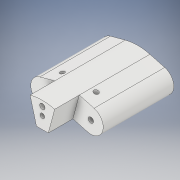
# Autodesk Inventor part: Body
Saved by Autodesk Inventor 2017 SP1 (Build 210196100, 196)
## iProperties
Created: 2018-02-11
Part Number: Body
Material: ABS Plastic
Document SubType Name: Modeling
Designer: Zach
Density: 1.06 g/cm^3
Appearance: CR White
Author: Zach
Autodesk Inventor part; units mm, degrees
ref_plane "YZ Plane" through (0, 0, 0) normal (1, 0, 0) x (0, 1, 0)
ref_plane "XZ Plane" through (0, 0, 0) normal (0, 1, 0) x (-1, 0, 0)
ref_plane "XY Plane" through (0, 0, 0) normal (0, 0, 1) x (1, 0, 0)
sketch "Sketch1" plane through (0, 0, 0) normal (0, 0, 1) x (1, 0, 0)
  circle A0 centre (31.1774, 0) radius 8 construction
  circle A1 centre (0, 0) radius 8 construction
  line L0 (7.5887, 10.3156) -> (11.7298, -5.1392) construction
  line L1 (11.7298, -5.1392) -> (2.0706, -7.7274)
  line L2 (-2.0706, 7.7274) -> (7.5887, 10.3156)
  line L3 (19.4476, -5.1392) -> (23.5887, 10.3156) construction
  line L4 (23.5887, 10.3156) -> (33.248, 7.7274)
  line L5 (19.4476, -5.1392) -> (29.1069, -7.7274)
  line L6 (7.5887, 10.3156) -> (23.5887, 10.3156) construction
  line L7 (11.7298, -5.1392) -> (19.4476, -5.1392)
  arc A2 (-2.0706, 7.7274) -> (2.0706, -7.7274) centre (0, 0) ccw
  arc A3 (29.1069, -7.7274) -> (33.248, 7.7274) centre (31.1774, 0) ccw
  arc A4 (23.5887, 10.3156) -> (7.5887, 10.3156) centre (15.5887, -19.5408) ccw
  point P0 (15.5887, 10.3156)
  dimension "d0" = 16
  dimension "d1" = 16
  dimension "d2" = 16
  dimension "d3" = 10
  dimension "d4" = 10
  dimension "d5" = 16
  dimension "d6" = 16
  dimension "d7" = 75
  constraints: 16 end point, 10 point on circle, 10 tangent, 5 centre point, 2 horizontal alignment, 2 perpendicular, 1 coincident, 1 horizontal, 1 midpoint, 1 point on line
  measures "d0" diameter of A0
  measures "d1" diameter of A1
  measures "d2" distance of L0.start L7.start
  measures "d3" distance from line of A1.centre L0
  measures "d4" distance from line of L3 A0.centre
  measures "d5" distance of L5.start L3.end
  measures "d6" distance of L0.start L3.end
  measures "d7" angle of L6 L0
extrude "Extrusion1" add sketch "Sketch1" along normal blind 46
sketch "Sketch2" plane through (0, 0, 46) normal (0, 0, 1) x (1, 0, 0)
  arc A0 (-2.0706, 7.7274) -> (2.0706, -7.7274) centre (0, 0) ccw projected
  arc A1 (29.1069, -7.7274) -> (33.248, 7.7274) centre (31.1774, 0) ccw projected
  line L0 (11.7298, -5.1392) -> (19.4476, -5.1392) projected
  circle A2 centre (0, 0) radius 1.75
  circle A3 centre (31.1774, 0) radius 1.75
  circle A4 centre (15.5887, 7.8608) radius 1.75
  point P0 (0, 0)
  point P1 (15.5887, -5.1392)
  dimension "d11" = 3.5
  dimension "d12" = 3.5
  dimension "d13" = 3.5
  dimension "d14" = 13
  constraints: 3 centre point, 2 coincident, 1 midpoint, 1 vertical alignment
  measures "d11" diameter of A2
  measures "d12" diameter of A3
  measures "d13" diameter of A4
  measures "d14" distance from line of L0 A4.centre
extrude "Extrusion2" cut sketch "Sketch2" against normal through all
sketch "Sketch3" plane through (0, 0, 46) normal (0, 0, 1) x (1, 0, 0)
  arc A0 (23.5887, 10.3156) -> (7.5887, 10.3156) centre (15.5887, -19.5408) ccw projected
  line L0 (7.5887, 10.3156) -> (23.5887, 10.3156)
  line L1 (19.4476, -5.1392) -> (29.1069, -7.7274) projected
  line L2 (23.5887, 10.3156) -> (19.4476, -5.1392)
  line L3 (11.7298, -5.1392) -> (19.4476, -5.1392) projected
  line L4 (19.4476, -5.1392) -> (11.7298, -5.1392)
  line L5 (11.7298, -5.1392) -> (7.5887, 10.3156)
  circle A1 centre (15.5887, 7.8608) radius 1.75 projected
  point P0 (0, 0)
  constraints: 8 end point, 1 collinear, 1 horizontal, 1 perpendicular
extrude "Extrusion3" add sketch "Sketch3" along normal blind 16
sketch "Sketch4" plane through (0, 0, 62) normal (0, 0, 1) x (1, 0, 0)
  arc A0 (23.5887, 10.3156) -> (7.5887, 10.3156) centre (15.5887, -19.5408) ccw construction
  line L0 (7.5887, 10.3156) -> (23.5887, 10.3156) construction
  line L1 (23.5887, 10.3156) -> (15.5887, 10.3156) construction
  line L2 (11.7298, -5.1392) -> (19.4476, -5.1392) construction
  line L3 (15.5887, -5.1392) -> (15.5887, 10.3156) construction
  circle A1 centre (15.5887, 2.5882) radius 1.5
  point P0 (0, 0)
  dimension "d19" = 3
  constraints: 6 end point, 3 midpoint, 1 centre point, 1 horizontal, 1 perpendicular
  measures "d19" diameter of A1
extrude "Extrusion4" cut sketch "Sketch4" against normal through all
sketch "Sketch7" plane through (0, 0, 0) normal (0, 1, 0) x (-1, 0, 0)
  circle A0 centre (-26.5887, 38) radius 1.5
  circle A1 centre (-4.5887, 38) radius 1.5
  line L0 (-7.5887, 62) -> (-23.5887, 62) construction
  line L1 (-26.5887, 38) -> (-4.5887, 38) construction
  point P0 (0, 0)
  point P1 (-15.5887, 62)
  point P2 (-15.5887, 38)
  dimension "d28" = 3
  dimension "d29" = 3
  dimension "d30" = 22
  dimension "d31" = 24
  constraints: 2 centre point, 2 end point, 2 midpoint, 1 horizontal, 1 vertical alignment
  measures "d28" diameter of A0
  measures "d29" diameter of A1
  measures "d30" distance of L1.start L1.end
  measures "d31" distance between parallel lines of L1 L0
extrude "Extrusion7" cut sketch "Sketch7" along normal through all
body "Solid1"
